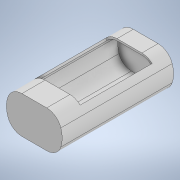
# Autodesk Inventor part: Корпус
Saved by Autodesk Inventor 2022.1 (Build 261234000, 234)
## iProperties
Created: 2021-12-23
Part Number: Корпус
Material: Типовые
Document SubType Name: Modeling
Designer: Grigori
Density: 1 g/cm^3
Appearance: По умолчанию
Author: Grigori
Autodesk Inventor part; units mm, degrees
ref_plane "YZ Plane" through (0, 0, 0) normal (1, 0, 0) x (0, 1, 0)
ref_plane "XZ Plane" through (0, 0, 0) normal (0, 1, 0) x (-1, 0, 0)
ref_plane "XY Plane" through (0, 0, 0) normal (0, 0, 1) x (1, 0, 0)
sketch "Эскиз1" plane through (0, 0, 0) normal (0, 0, 1) x (1, 0, 0)
  line L0 (-75, 100) -> (75, 100)
  line L1 (75, -100) -> (-75, -100)
  line L2 (-110, 100) -> (-75, 100)
  line L3 (-150, 0) -> (-110, 0) construction
  line L4 (-110, -100) -> (-75, -100)
  arc A0 (-110, 100) -> (-110, -100) centre (-5, 0) ccw
  arc A1 (110, -100) -> (110, 100) centre (5, 0) ccw
  line L5 (75, 100) -> (110, 100)
  line L6 (75, -100) -> (110, -100)
  point P0 (0, 0)
  constraints: 14 end point, 5 point on circle, 3 horizontal, 2 centre point, 2 parallel
extrude "Выдавливание1" add sketch "Эскиз1" against normal blind 600
fillet "Сопряжение1" radius 80 1 edges at (-110, 100, -300)
fillet "Сопряжение2" radius 80 3 edges at (110, 100, -300) (110, -100, -300) (-110, -100, -300)
shell "Оболочка1" thickness 10 removed faces 1 at (-22.2822, 33.3333, 0)
sketch "Эскиз2" plane through (0, 0, 0) normal (0, 0, 1) x (1, 0, 0)
  line L0 (66.8466, 100) -> (-66.8466, 100) projected
  arc A0 (-66.8466, 100) -> (-142.9655, 44.6154) centre (-66.8466, 20) ccw projected
  arc A1 (-142.9655, 44.6154) -> (-142.9655, -44.6154) centre (-5, 0) ccw projected
  arc A2 (-142.9655, -44.6154) -> (-66.8466, -100) centre (-66.8466, -20) ccw projected
  line L1 (-66.8466, -100) -> (66.8466, -100) projected
  arc A3 (66.8466, -100) -> (142.9655, -44.6154) centre (66.8466, -20) ccw projected
  arc A4 (142.9655, -44.6154) -> (142.9655, 44.6154) centre (5, 0) ccw projected
  arc A5 (142.9655, 44.6154) -> (66.8466, 100) centre (66.8466, 20) ccw projected
  point P0 (0, 0)
extrude "Выдавливание2" add sketch "Эскиз2" against normal blind 10
sketch "Эскиз3" plane through (-66.8466, 100, 0) normal (0, 1, 0) x (1, 0, 0)
  line L0 (-55.0683, 512.598) -> (188.7615, 512.598)
  line L1 (188.7615, 512.598) -> (188.7615, 125.0142)
  line L2 (188.7615, 125.0142) -> (-55.0683, 125.0142)
  line L3 (-55.0683, 125.0142) -> (-55.0683, 512.598)
  line L4 (-55.0683, 512.598) -> (188.7615, 125.0142) construction
  line L5 (188.7615, 512.598) -> (-55.0683, 125.0142) construction
  point P0 (66.8466, 0)
  point P1 (66.8466, 318.8061)
  constraints: 12 end point, 2 midpoint, 2 parallel, 1 horizontal, 1 perpendicular
extrude "Выдавливание3" cut sketch "Эскиз3" against normal blind 56
